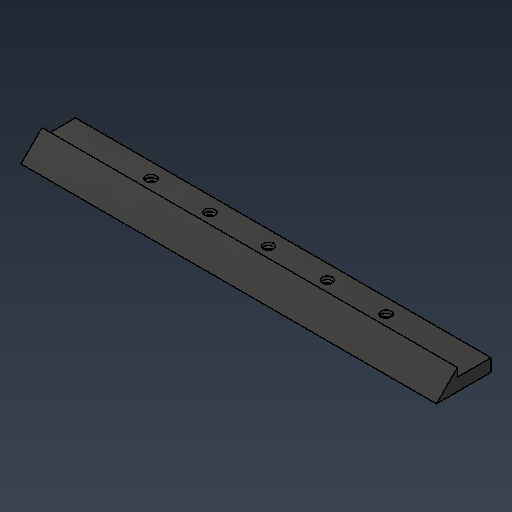
# Autodesk Inventor part: Plog2
Saved by Autodesk Inventor 2026.2 (Build 302298010, 298A)
## iProperties
Created: 2022-01-27
Part Number: Plog2
Material: Steel, High Strength, Low Alloy
Document SubType Name: Modeling
Designer: Michał
Density: 7.85 g/cm^3
Appearance: Dark Gray
Mass: 26.5441 g
Surface Area: 33.9759 cm^2
Volume: 3.38142 cm^3
Author: Michał
Autodesk Inventor part; units mm, degrees
ref_plane "YZ Plane" through (0, 0, 0) normal (1, 0, 0) x (0, 1, 0)
ref_plane "XZ Plane" through (0, 0, 0) normal (0, 1, 0) x (-1, 0, 0)
ref_plane "XY Plane" through (0, 0, 0) normal (0, 0, 1) x (1, 0, 0)
sketch "Szkic1" plane through (0, 0, 0) normal (1, 0, 0) x (0, 1, 0)
  line L0 (0, 0) -> (3, -3)
  line L1 (3, -3) -> (3, -13)
  line L2 (3, -13) -> (0, -13)
  line L3 (0, -13) -> (0, -3)
  line L4 (0, -3) -> (0, 0)
  line L5 (0, -3) -> (3, -3)
  line L6 (3, -3) -> (5, -5)
  line L7 (5, -5) -> (3, -5)
  dimension "d1" = 3
  dimension "d2" = 45
  dimension "d43" = 2
  dimension "d44" = 45
  dimension "d45" = 3
  dimension "d46" = 10
  constraints: 16 end point, 4 perpendicular, 1 point on line, 1 vertical
  measures "d1" distance between parallel lines of L4 L1
  measures "d2" angle of L4 L0
  measures "d43" distance of L6.end L7.end
  measures "d44" angle of L7 L6
  measures "d45" distance of L3.end L0.start
  measures "d46" distance of L2.end L3.end
extrude "Wyciągnięcie proste1" add sketch "Szkic1" along normal blind 99
sketch "Sketch4" plane through (0, 0, -13) normal (0, -1, 0) x (1, 0, 0)
  line L0 (0, 0) -> (0, 13) projected
  line L1 (0, 0) -> (99, 0) projected
  line L2 (99, 13) -> (99, 0) projected
  line L3 (0, 13) -> (99, 13) projected
  line L4 (81, 0) -> (81, 13)
  line L5 (0, 13) -> (99, 13) projected
  line L6 (18, 13) -> (18, 0)
  circle A0 centre (77.5, 3.5) radius 3.5
  circle A1 centre (63.5, 3.5) radius 3.5
  circle A2 centre (35.5, 3.5) radius 3.5
  circle A3 centre (21.5, 3.5) radius 3.5
  line L7 (0, 0) -> (99, 0) projected
  circle A4 centre (49.5, 3.5) radius 3.5
  dimension "d22" = 18
  dimension "d23" = 18
  dimension "d24" = 7
  dimension "d25" = 7
  dimension "d26" = 7
  dimension "d27" = 7
  dimension "d28" = 7
  dimension "d30" = 14
  dimension "d31" = 14
  dimension "d32" = 14
  dimension "d33" = 14
  constraints: 7 tangent, 5 centre point, 4 end point, 4 point on line, 2 perpendicular
  measures "d22" distance between parallel lines of L2 L4
  measures "d23" distance between parallel lines of L0 L6
  measures "d24" diameter of A0
  measures "d25" diameter of A1
  measures "d26" diameter of A2
  measures "d27" diameter of A3
  measures "d28" diameter of A4
  measures "d30" distance of A1.centre A0.centre
  measures "d31" distance of A4.centre A1.centre
  measures "d32" distance of A2.centre A4.centre
  measures "d33" distance of A3.centre A2.centre
hole "Hole2" at (77.5, 0, -9.5) at (63.5, 0, -9.5) at (49.5, 0, -9.5) at (35.5, 0, -9.5) at (21.5, 0, -9.5) direction (0, 1, 0) diameter 2.459 depth 8.8 countersink diameter 7 countersink angle 90 thread size "M3x0.5" class "6H" standard "ISO Metric profile"
equation "\"d23\" = d22"
equation "\"d30\" = d33"
equation "\"d31\" = d33"
equation "\"d32\" = d33"
